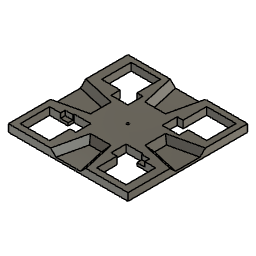
base+plate+radial (Autodesk Fusion 360 design; units mm, degrees)
Autodesk Fusion 360 part; units mm, degrees
note: some values were not read from the file. Set by a fixed rule: which sketch regions a step uses.
sketch "Sketch1" plane through (0, 0, 0) normal (0, 0, 1) x (1, 0, 0)
  line L0 (0, 0) -> (10, 0)
  line L1 (10, 0) -> (101.6, 0)
  line L2 (101.6, 0) -> (101.6, 101.6)
  line L3 (101.6, 101.6) -> (0, 101.6)
  line L4 (0, 101.6) -> (0, 0)
  dimension "d32" = 101.6
  dimension "d55" = 101.6
  dimension "d56" = 101.6
  constraint coincident L0.start L4.end
  constraint horizontal L0
  constraint parallel L0 L1
  constraint perpendicular L1 L2
  constraint perpendicular L2 L3
  constraint perpendicular L0 L4
  measures "d32" distance of L0.start L1.end
  measures "d55" distance of L0.start L3.end
  measures "d56" distance of L1.end L2.end
extrude "Extrude1" add sketch "Sketch1" along normal blind 6.35
sketch "Sketch2" plane through (0, 0, 6.35) normal (0, 0, 1) x (-1, 0, 0)
  line L0 (0, -101.6) -> (0, 0)
  line L1 (0, 0) -> (-101.6, 0)
  line L2 (-101.6, 0) -> (-101.6, -101.6)
  line L3 (-101.6, -101.6) -> (0, -101.6)
  line L4 (0, 0) -> (-50.8, 0)
  line L5 (0, 0) -> (0, -50.8)
  circle A0 centre (-50.8, -50.8) radius 1
  line L6 (0, -50.8) -> (-49.8, -50.8)
  line L7 (-51.8, -50.8) -> (-101.6, -50.8)
  line L8 (-50.8, 0) -> (-50.8, -49.8)
  line L9 (-50.8, -51.8) -> (-50.8, -101.6)
  dimension "d33" = 50.8
  dimension "d34" = 50.8
  dimension "d35" = 2
  constraint coincident L0.end L1.start
  constraint perpendicular L0 L4
  constraint midpoint L3 L9.end
  constraint perpendicular L1 L5
  constraint midpoint L2 L7.end
  constraint coincident A0 L6.end
  constraint collinear L6 L7
  constraint coincident A0.centre L6
  constraint coincident A0 L7.start
  constraint coincident A0 L8.end
  constraint coincident A0 L9.start
  constraint collinear L8 L9
  measures "d33" distance of L0.end L4.end
  measures "d34" distance of L0.end L5.end
  measures "d35" diameter of A0
extrude "Extrude2" cut sketch "Sketch2" against normal blind 6.35 contours A0
sketch "Sketch3" plane through (0, 0, 6.35) normal (0, 0, 1) x (-1, 0, 0)
  line L0 (0, -101.6) -> (0, 0)
  line L1 (0, 0) -> (-101.6, 0)
  line L2 (-101.6, 0) -> (-101.6, -101.6)
  line L3 (-101.6, -101.6) -> (0, -101.6)
  line L4 (0, -50.8) -> (0, -38.1)
  line L5 (0, -50.8) -> (0, -63.5)
  line L6 (-50.8, -101.6) -> (-38.1, -101.6)
  line L7 (-50.8, -101.6) -> (-63.5, -101.6)
  line L8 (-101.6, -50.8) -> (-101.6, -63.5)
  line L9 (-101.6, -50.8) -> (-101.6, -38.1)
  line L10 (-50.8, 0) -> (-38.1, 0)
  line L11 (-50.8, 0) -> (-63.5, 0)
  line L12 (-50.8019, -76.2) -> (-43.8829, -76.2)
  line L13 (-50.8019, -76.2) -> (-57.7209, -76.2)
  line L14 (-25.4, -50.8) -> (-25.4, -43.881)
  line L15 (-25.4, -50.8) -> (-25.4, -57.719)
  line L16 (-76.2, -50.7996) -> (-76.2, -57.7186)
  line L17 (-76.2, -50.7996) -> (-76.2, -43.8806)
  line L18 (-38.1, 0) -> (-43.881, -25.4)
  line L19 (-63.5, 0) -> (-57.719, -25.4)
  line L20 (0, -38.1) -> (-25.4, -43.881)
  line L21 (0, -63.5) -> (-25.4, -57.719)
  line L22 (-38.1, -101.6) -> (-43.8829, -76.2)
  line L23 (-63.5, -101.6) -> (-57.7209, -76.2)
  line L24 (-101.6, -63.5) -> (-76.2, -57.7186)
  line L25 (-101.6, -38.1) -> (-76.2, -43.8806)
  circle A0 centre (-50.8, -50.8) radius 1
  line L26 (-50.8, -25.4) -> (-43.881, -25.4)
  line L27 (-50.8, -25.4) -> (-57.719, -25.4)
  dimension "d8" = 12.7
  dimension "d9" = 12.7
  dimension "d10" = 12.7
  dimension "d11" = 12.7
  dimension "d12" = 12.7
  dimension "d13" = 12.7
  dimension "d14" = 12.7
  dimension "d15" = 12.7
  dimension "d17" = 25.4
  dimension "d18" = 25.4
  dimension "d36" = 6.919
  dimension "d37" = 6.919
  dimension "d40" = 6.919
  dimension "d41" = 6.919
  dimension "d42" = 25.4
  dimension "d43" = 26.0496
  dimension "d44" = 26.0496
  dimension "d45" = 26.0496
  dimension "d46" = 6.919
  dimension "d47" = 6.919
  dimension "d48" = 6.919
  dimension "d49" = 6.919
  dimension "d50" = 25.4
  dimension "d51" = 25.4
  dimension "d52" = 26.05
  constraint midpoint L1 L10.start
  constraint midpoint L2 L8.start
  constraint midpoint L3 L6.start
  constraint midpoint L0 L4.start
  constraint horizontal L10
  constraint horizontal L27
  constraint horizontal L26
  constraint vertical L16
  constraint vertical L17
  constraint horizontal L12
  constraint horizontal L13
  constraint horizontal L6
  constraint vertical L5
  constraint vertical L4
  constraint vertical L15
  constraint vertical L14
  constraint horizontal L11
  constraint horizontal L7
  constraint vertical L8
  constraint vertical L9
  measures "d8" distance of L4.start L4.end
  measures "d9" distance of L4.start L5.end
  measures "d10" distance of L6.start L6.end
  measures "d11" distance of L6.start L7.end
  measures "d12" distance of L8.start L8.end
  measures "d13" distance of L8.start L9.end
  measures "d14" distance of L10.start L10.end
  measures "d15" distance of L10.start L11.end
  measures "d17" distance of L8.start L16.start
  measures "d18" distance of L4.start L14.start
  measures "d36" distance of L14.start L15.end
  measures "d37" distance of L14.start L14.end
  measures "d40" horizontal distance of L18.end L26.start
  measures "d41" horizontal distance of L19.end L26.start
  measures "d42" distance of L10.start L26.start
  measures "d43" distance of L4.end L14.end
  measures "d44" distance of L10.end L18.end
  measures "d45" distance of L11.end L19.end
  measures "d46" distance of L16.start L16.end
  measures "d47" distance of L16.start L17.end
  measures "d48" distance of L12.start L12.end
  measures "d49" distance of L12.start L13.end
  measures "d50" vertical distance of L6.start L12.start
  measures "d51" horizontal distance of L8.start L16.start
  measures "d52" distance of L6.end L12.end
extrude "Extrude3" cut sketch "Sketch3" against normal blind 4.445 contours L0 L4 L5 L14 L15 L20 L21 | L3 L6 L7 L12 L13 L22 L23 | L1 L10 L11 L18 L19 L26 L27 | L2 L8 L9 L16 L17 L24 L25
chamfer "Chamfer1" distance 2.2225 angle 45 6 edges at (40.9905, 12.7, 6.35) (40.9905, 12.7, 1.905) (60.6095, 12.7, 6.35) (60.6095, 12.7, 1.905) (50.8, 25.4, 1.905) (50.8, 25.4, 6.35) measured on face at (23.0943, 78.5063, 6.35) measured on face at (40.027, 8.4667, 4.8683) measured on face at (23.0943, 78.5063, 6.35) measured on face at (61.573, 8.4667, 4.8683) measured on face at (53.1063, 25.4, 4.8683) measured on face at (23.0943, 78.5063, 6.35)
chamfer "Chamfer2" distance 2.2225 angle 45 6 edges at (88.9, 60.6093, 1.905) (88.9, 60.6093, 6.35) (76.2, 50.7996, 6.35) (76.2, 50.7996, 1.905) (88.9, 40.9903, 6.35) (88.9, 40.9903, 1.905) measured on face at (93.1333, 61.5729, 4.8683) measured on face at (14.036, 21.9074, 6.35) measured on face at (14.036, 21.9074, 6.35) measured on face at (76.2, 53.1059, 4.8683) measured on face at (14.036, 21.9074, 6.35) measured on face at (93.1333, 40.0269, 4.8683)
chamfer "Chamfer3" distance 2.2225 angle 45 6 edges at (60.6105, 88.9, 6.35) (60.6105, 88.9, 1.905) (50.8019, 76.2, 6.35) (50.8019, 76.2, 1.905) (40.9915, 88.9, 6.35) (40.9915, 88.9, 1.905) measured on face at (79.6926, 87.5639, 6.35) measured on face at (61.5736, 93.1333, 4.8683) measured on face at (79.6926, 87.5639, 6.35) measured on face at (48.4956, 76.2, 4.8683) measured on face at (79.6926, 87.5639, 6.35) measured on face at (40.0276, 93.1333, 4.8683)
chamfer "Chamfer4" distance 2.2225 angle 45 6 edges at (12.7, 60.6095, 1.905) (12.7, 60.6095, 6.35) (25.4, 50.8, 6.35) (25.4, 50.8, 1.905) (12.7, 40.9905, 6.35) (12.7, 40.9905, 1.905) measured on face at (16.9333, 59.646, 3.3867) measured on face at (14.0366, 79.6926, 6.35) measured on face at (14.0366, 79.6926, 6.35) measured on face at (25.4, 48.4937, 4.8683) measured on face at (14.0366, 79.6926, 6.35) measured on face at (8.4667, 40.027, 4.8683)
sketch "Sketch5" plane through (0, 0, 6.35) normal (0, 0, 1) x (-1, 0, 0)
  line L0 (0, -65.7793) -> (-27.6225, -59.4925)
  line L1 (-27.6225, -59.4925) -> (-27.6225, -42.1075)
  line L2 (-27.6225, -42.1075) -> (0, -35.8207)
  line L3 (0, -35.8207) -> (0, 0)
  line L4 (0, 0) -> (-35.8207, 0)
  line L5 (-35.8207, 0) -> (-42.1075, -27.6225)
  line L6 (-42.1075, -27.6225) -> (-59.4925, -27.6225)
  line L7 (-59.4925, -27.6225) -> (-65.7793, 0)
  line L8 (-65.7793, 0) -> (-101.6, 0)
  line L9 (-101.6, 0) -> (-101.6, -35.8207)
  line L10 (-101.6, -35.8207) -> (-73.9775, -42.1071)
  line L11 (-73.9775, -42.1071) -> (-73.9775, -59.4921)
  line L12 (-73.9775, -59.4921) -> (-101.6, -65.7793)
  line L13 (-101.6, -65.7793) -> (-101.6, -101.6)
  line L14 (-101.6, -101.6) -> (-65.7793, -101.6)
  line L15 (-65.7793, -101.6) -> (-59.4946, -73.9775)
  line L16 (-59.4946, -73.9775) -> (-42.1096, -73.9775)
  line L17 (-42.1096, -73.9775) -> (-35.8206, -101.6)
  line L18 (-35.8206, -101.6) -> (0, -101.6)
  line L19 (0, -101.6) -> (0, -65.7793)
  circle A0 centre (-50.8, -50.8) radius 1
  line L20 (-5, -30) -> (-20.7125, -30)
  line L21 (-30, -22.3) -> (-30, -5)
  line L22 (-30, -5) -> (-5, -5)
  line L23 (-5, -5) -> (-5, -30)
  line L24 (-6.9943, -97.2437) -> (-31.9943, -97.2437)
  line L25 (-31.9943, -97.2437) -> (-31.9943, -77.2437)
  line L26 (-22.7063, -72.2437) -> (-6.9943, -72.2437)
  line L27 (-6.9943, -72.2437) -> (-6.9943, -97.2437)
  line L28 (-71.6399, -96.8328) -> (-96.6399, -96.8328)
  line L29 (-96.6399, -96.8328) -> (-96.6399, -71.8328)
  line L30 (-96.6399, -71.8328) -> (-80.9279, -71.8328)
  line L31 (-71.6399, -76.8328) -> (-71.6399, -96.8328)
  line L32 (-70, -5) -> (-95, -5)
  line L33 (-95, -5) -> (-95, -30)
  line L34 (-95, -30) -> (-79.288, -30)
  line L35 (-70, -22.3) -> (-70, -5)
  line L36 (-65, -35) -> (-79.288, -35)
  line L37 (-79.288, -35) -> (-79.288, -30)
  line L38 (-70, -22.3) -> (-65, -22.3)
  line L39 (-65, -22.3) -> (-65, -35)
  line L40 (-35, -35) -> (-20.7125, -35)
  line L41 (-20.7125, -35) -> (-20.7125, -30)
  line L42 (-30, -22.3) -> (-35, -22.3)
  line L43 (-35, -22.3) -> (-35, -35)
  line L44 (-31.9943, -77.2437) -> (-36.9943, -77.2437)
  line L45 (-36.9943, -77.2437) -> (-36.9943, -64.5437)
  line L46 (-36.9943, -64.5437) -> (-22.7063, -64.5437)
  line L47 (-22.7063, -64.5437) -> (-22.7063, -72.2437)
  line L48 (-71.6399, -76.8328) -> (-66.6399, -76.8328)
  line L49 (-66.6399, -76.8328) -> (-66.6399, -64.1328)
  line L50 (-66.6399, -64.1328) -> (-80.9279, -64.1328)
  line L51 (-80.9279, -64.1328) -> (-80.9279, -71.8328)
  line L52 (-35, -35) -> (-20.7125, -35)
  line L53 (-20.7125, -35) -> (-20.7125, -30)
  line L54 (-30, -22.3) -> (-35, -22.3)
  line L55 (-35, -22.3) -> (-35, -35)
  dimension "d57" = 14.2875
  dimension "d58" = 12.7
  dimension "d59" = 14.2875
  dimension "d60" = 12.7
  dimension "d61" = 14.288
  dimension "d62" = 12.7
  dimension "d63" = 14.288
  dimension "d64" = 12.7
  dimension "d65" = 12.7
  dimension "d66" = 14.288
  constraint horizontal L20
  constraint vertical L21
  constraint horizontal L22
  constraint vertical L23
  constraint horizontal L24
  constraint vertical L25
  constraint horizontal L26
  constraint vertical L27
  constraint horizontal L28
  constraint vertical L29
  constraint horizontal L30
  constraint vertical L31
  constraint horizontal L32
  constraint vertical L33
  constraint horizontal L34
  constraint vertical L35
  constraint horizontal L36
  constraint vertical L37
  constraint horizontal L38
  constraint vertical L39
  constraint horizontal L40
  constraint vertical L41
  constraint horizontal L42
  constraint vertical L43
  constraint horizontal L44
  constraint vertical L45
  constraint horizontal L46
  constraint vertical L47
  constraint horizontal L48
  constraint vertical L49
  constraint horizontal L50
  constraint vertical L51
  constraint horizontal L52
  constraint vertical L53
  constraint horizontal L54
  constraint vertical L55
  measures "d57" distance of L40.start L40.end
  measures "d58" distance of L40.start L42.end
  measures "d59" distance of L40.start L40.end
  measures "d60" distance of L40.start L42.end
  measures "d61" distance of L36.start L36.end
  measures "d62" distance of L36.start L38.end
  measures "d63" distance of L45.end L46.end
  measures "d64" distance of L44.end L45.end
  measures "d65" distance of L48.end L49.end
  measures "d66" distance of L49.end L50.end
extrude "Extrude5" cut sketch "Sketch5" against normal blind 6.35 contours L20 L21 L22 L23 L40 L41 L42 L43 L52 L53 L54 L55 | L24 L25 L26 L27 L44 L45 L46 L47 | L28 L29 L30 L31 L48 L49 L50 L51 | L32 L33 L34 L35 L36 L37 L38 L39
sketch "Sketch6" plane through (0, 0, 6.35) normal (0, 0, 1) x (-1, 0, 0)
  line L0 (-35, -35) -> (-35, -22.3)
  line L1 (-35, -22.3) -> (-30, -22.3)
  line L2 (-30, -22.3) -> (-30, -5)
  line L3 (-30, -5) -> (-5, -5)
  line L4 (-5, -5) -> (-5, -30)
  line L5 (-5, -30) -> (-20.7125, -30)
  line L6 (-20.7125, -30) -> (-20.7125, -35)
  line L7 (-20.7125, -35) -> (-35, -35)
  line L8 (-66.6399, -64.1328) -> (-66.6399, -76.8328)
  line L9 (-66.6399, -76.8328) -> (-71.6399, -76.8328)
  line L10 (-71.6399, -76.8328) -> (-71.6399, -96.8328)
  line L11 (-71.6399, -96.8328) -> (-96.6399, -96.8328)
  line L12 (-96.6399, -96.8328) -> (-96.6399, -71.8328)
  line L13 (-96.6399, -71.8328) -> (-80.9279, -71.8328)
  line L14 (-80.9279, -71.8328) -> (-80.9279, -64.1328)
  line L15 (-80.9279, -64.1328) -> (-66.6399, -64.1328)
  line L16 (-36.9943, -77.2437) -> (-36.9943, -64.5437)
  line L17 (-36.9943, -64.5437) -> (-22.7063, -64.5437)
  line L18 (-22.7063, -64.5437) -> (-22.7063, -72.2437)
  line L19 (-22.7063, -72.2437) -> (-6.9943, -72.2437)
  line L20 (-6.9943, -72.2437) -> (-6.9943, -97.2437)
  line L21 (-6.9943, -97.2437) -> (-31.9943, -97.2437)
  line L22 (-31.9943, -97.2437) -> (-31.9943, -77.2437)
  line L23 (-31.9943, -77.2437) -> (-36.9943, -77.2437)
  line L24 (-95, -5) -> (-70, -5)
  line L25 (-70, -5) -> (-70, -22.3)
  line L26 (-70, -22.3) -> (-65, -22.3)
  line L27 (-65, -22.3) -> (-65, -35)
  line L28 (-65, -35) -> (-79.288, -35)
  line L29 (-79.288, -35) -> (-79.288, -30)
  line L30 (-79.288, -30) -> (-95, -30)
  line L31 (-95, -30) -> (-95, -5)
  line L32 (0, -65.7793) -> (-27.6225, -59.4925)
  line L33 (-27.6225, -59.4925) -> (-27.6225, -42.1075)
  line L34 (-27.6225, -42.1075) -> (0, -35.8207)
  line L35 (0, -35.8207) -> (0, 0)
  line L36 (0, 0) -> (-35.8207, 0)
  line L37 (-35.8207, 0) -> (-42.1075, -27.6225)
  line L38 (-42.1075, -27.6225) -> (-59.4925, -27.6225)
  line L39 (-59.4925, -27.6225) -> (-65.7793, 0)
  line L40 (-65.7793, 0) -> (-101.6, 0)
  line L41 (-101.6, 0) -> (-101.6, -35.8207)
  line L42 (-101.6, -35.8207) -> (-73.9775, -42.1071)
  line L43 (-73.9775, -42.1071) -> (-73.9775, -59.4921)
  line L44 (-73.9775, -59.4921) -> (-101.6, -65.7793)
  line L45 (-101.6, -65.7793) -> (-101.6, -101.6)
  line L46 (-101.6, -101.6) -> (-65.7793, -101.6)
  line L47 (-65.7793, -101.6) -> (-59.4946, -73.9775)
  line L48 (-59.4946, -73.9775) -> (-42.1096, -73.9775)
  line L49 (-42.1096, -73.9775) -> (-35.8206, -101.6)
  line L50 (-35.8206, -101.6) -> (0, -101.6)
  line L51 (0, -101.6) -> (0, -65.7793)
  circle A0 centre (-50.8, -50.8) radius 1
  line L52 (-70, -22.3) -> (-66, -22.3)
  line L53 (-66, -22.3) -> (-66, -15.8)
  line L54 (-66, -15.8) -> (-70, -15.8)
  line L55 (-70, -22.3) -> (-70, -15.8)
  line L56 (-30, -22.3) -> (-34, -22.3)
  line L57 (-34, -22.3) -> (-34, -15.8)
  line L58 (-34, -15.8) -> (-30, -15.8)
  line L59 (-30, -22.3) -> (-30, -15.8)
  dimension "d67" = 4
  dimension "d68" = 6.5
  dimension "d69" = 4
  dimension "d70" = 6.5
  constraint coincident L25.end L26.start
  constraint perpendicular L25 L52
  constraint perpendicular L26 L53
  constraint coincident L25 L54.end
  constraint perpendicular L25 L54
  constraint coincident L1.end L2.start
  constraint perpendicular L2 L56
  constraint perpendicular L1 L57
  constraint coincident L2 L58.end
  constraint perpendicular L2 L58
  measures "d67" distance of L25.end L52.end
  measures "d68" distance of L52.end L53.end
  measures "d69" distance of L1.end L56.end
  measures "d70" distance of L56.end L57.end
sketch "Sketch7" plane through (0, 0, 6.35) normal (0, 0, 1) x (-1, 0, 0)
  circle A0 centre (-50.8, -50.8) radius 1
  line L0 (0, -65.7793) -> (-27.6225, -59.4925)
  line L1 (-27.6225, -59.4925) -> (-27.6225, -42.1075)
  line L2 (-27.6225, -42.1075) -> (0, -35.8207)
  line L3 (0, -35.8207) -> (0, 0)
  line L4 (0, 0) -> (-35.8207, 0)
  line L5 (-35.8207, 0) -> (-42.1075, -27.6225)
  line L6 (-42.1075, -27.6225) -> (-59.4925, -27.6225)
  line L7 (-59.4925, -27.6225) -> (-65.7793, 0)
  line L8 (-65.7793, 0) -> (-101.6, 0)
  line L9 (-101.6, 0) -> (-101.6, -35.8207)
  line L10 (-101.6, -35.8207) -> (-73.9775, -42.1071)
  line L11 (-73.9775, -42.1071) -> (-73.9775, -59.4921)
  line L12 (-73.9775, -59.4921) -> (-101.6, -65.7793)
  line L13 (-101.6, -65.7793) -> (-101.6, -101.6)
  line L14 (-101.6, -101.6) -> (-65.7793, -101.6)
  line L15 (-65.7793, -101.6) -> (-59.4946, -73.9775)
  line L16 (-59.4946, -73.9775) -> (-42.1096, -73.9775)
  line L17 (-42.1096, -73.9775) -> (-35.8206, -101.6)
  line L18 (-35.8206, -101.6) -> (0, -101.6)
  line L19 (0, -101.6) -> (0, -65.7793)
  line L20 (-70, -22.3) -> (-65, -22.3)
  line L21 (-65, -22.3) -> (-65, -35)
  line L22 (-65, -35) -> (-79.288, -35)
  line L23 (-79.288, -35) -> (-79.288, -30)
  line L24 (-79.288, -30) -> (-95, -30)
  line L25 (-95, -30) -> (-95, -5)
  line L26 (-95, -5) -> (-70, -5)
  line L27 (-70, -5) -> (-70, -22.3)
  line L28 (-36.9943, -77.2437) -> (-36.9943, -64.5437)
  line L29 (-36.9943, -64.5437) -> (-22.7063, -64.5437)
  line L30 (-22.7063, -64.5437) -> (-22.7063, -72.2437)
  line L31 (-22.7063, -72.2437) -> (-6.9943, -72.2437)
  line L32 (-6.9943, -72.2437) -> (-6.9943, -97.2437)
  line L33 (-6.9943, -97.2437) -> (-31.9943, -97.2437)
  line L34 (-31.9943, -97.2437) -> (-31.9943, -77.2437)
  line L35 (-31.9943, -77.2437) -> (-36.9943, -77.2437)
  line L36 (-66.6399, -64.1328) -> (-66.6399, -76.8328)
  line L37 (-66.6399, -76.8328) -> (-71.6399, -76.8328)
  line L38 (-71.6399, -76.8328) -> (-71.6399, -96.8328)
  line L39 (-71.6399, -96.8328) -> (-96.6399, -96.8328)
  line L40 (-96.6399, -96.8328) -> (-96.6399, -71.8328)
  line L41 (-96.6399, -71.8328) -> (-80.9279, -71.8328)
  line L42 (-80.9279, -71.8328) -> (-80.9279, -64.1328)
  line L43 (-80.9279, -64.1328) -> (-66.6399, -64.1328)
  line L44 (-30, -22.3) -> (-30, -5)
  line L45 (-30, -5) -> (-5, -5)
  line L46 (-5, -5) -> (-5, -30)
  line L47 (-5, -30) -> (-20.7125, -30)
  line L48 (-20.7125, -30) -> (-20.7125, -35)
  line L49 (-20.7125, -35) -> (-35, -35)
  line L50 (-35, -35) -> (-35, -22.3)
  line L51 (-35, -22.3) -> (-30, -22.3)
  line L52 (-79.288, -30) -> (-85.788, -30)
  line L53 (-85.788, -30) -> (-85.788, -34)
  line L54 (-85.788, -34) -> (-79.288, -34)
  line L55 (-79.288, -30) -> (-79.288, -34)
  line L56 (-20.7125, -30) -> (-14.2125, -30)
  line L57 (-14.2125, -30) -> (-14.2125, -34)
  line L58 (-14.2125, -34) -> (-20.7125, -34)
  line L59 (-20.7125, -30) -> (-20.7125, -34)
  dimension "d73" = 6.5
  dimension "d74" = 4
  dimension "d75" = 6.5
  dimension "d76" = 4
  constraint coincident L23.end L24.start
  constraint perpendicular L23 L52
  constraint perpendicular L24 L53
  constraint coincident L23 L54.end
  constraint perpendicular L23 L54
  constraint coincident L47.end L48.start
  constraint perpendicular L48 L56
  constraint perpendicular L47 L57
  constraint coincident L48 L58.end
  constraint perpendicular L48 L58
  constraint perpendicular L58 L59
  measures "d73" distance of L23.end L52.end
  measures "d74" distance of L52.end L53.end
  measures "d75" distance of L47.end L56.end
  measures "d76" distance of L56.end L57.end
extrude "Extrude7" cut sketch "Sketch7" against normal blind 4 contours L23 L24 L52 L53 L54 L55 | L47 L48 L56 L57 L58 L59
